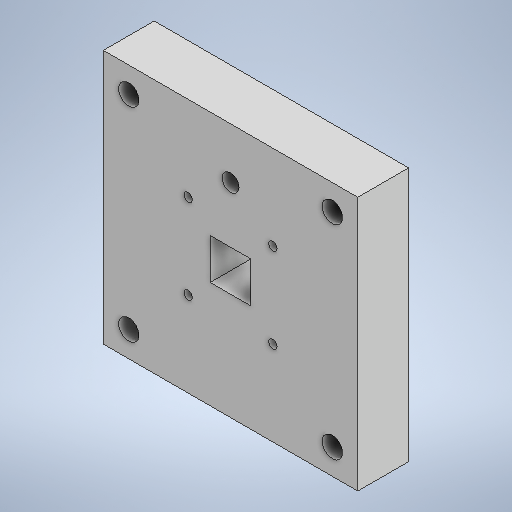
# Autodesk Inventor part: led_cnc
Saved by Autodesk Inventor 2025.1 (Build 291241000, 241)
## iProperties
Created: 2024-10-23
Part Number: led_cnc
Material: Ogólny
Document SubType Name: Modeling
Designer: PC
Density: 1 g/cm^3
Appearance: Domyślna
Author: PC
Autodesk Inventor part; units mm, degrees
ref_plane "YZ Plane" through (0, 0, 0) normal (1, 0, 0) x (0, 1, 0)
ref_plane "XZ Plane" through (0, 0, 0) normal (0, 1, 0) x (-1, 0, 0)
ref_plane "XY Plane" through (0, 0, 0) normal (0, 0, 1) x (1, 0, 0)
sketch "Szkic1" plane through (0, 0, 0) normal (0, 1, 0) x (-1, 0, 0)
  point P0 (0, 0)
sketch "Szkic2" plane through (0, 0, 0) normal (0, 0, 1) x (1, 0, 0)
  line L0 (-37.5, 37.5) -> (37.5, 37.5)
  line L1 (37.5, 37.5) -> (37.5, -37.5)
  line L2 (37.5, -37.5) -> (-37.5, -37.5)
  line L3 (-37.5, -37.5) -> (-37.5, 37.5)
  line L4 (-37.5, 37.5) -> (37.5, -37.5) construction
  line L5 (37.5, 37.5) -> (-37.5, -37.5) construction
  line L6 (-30, -30) -> (30, -30) construction
  line L7 (30, -30) -> (30, 30) construction
  line L8 (30, 30) -> (-30, 30) construction
  line L9 (-30, 30) -> (-30, -30) construction
  line L10 (-30, -30) -> (30, 30) construction
  line L11 (30, -30) -> (-30, 30) construction
  circle A0 centre (30, 30) radius 3
  circle A1 centre (30, -30) radius 3
  circle A2 centre (-30, 30) radius 3
  circle A3 centre (-30, -30) radius 3
  line L12 (-12.5, 12.5) -> (12.5, 12.5) construction
  line L13 (12.5, 12.5) -> (12.5, -12.5) construction
  line L14 (12.5, -12.5) -> (-12.5, -12.5) construction
  line L15 (-12.5, -12.5) -> (-12.5, 12.5) construction
  line L16 (-12.5, 12.5) -> (12.5, -12.5) construction
  line L17 (12.5, 12.5) -> (-12.5, -12.5) construction
  circle A4 centre (12.5, 12.5) radius 1.25
  circle A5 centre (12.5, -12.5) radius 1.25
  circle A6 centre (-12.5, -12.5) radius 1.25
  circle A7 centre (-12.5, 12.5) radius 1.25
  line L18 (-6, -6) -> (6, -6)
  line L19 (6, -6) -> (6, 6)
  line L20 (6, 6) -> (-6, 6)
  line L21 (-6, 6) -> (-6, -6)
  line L22 (-6, -6) -> (6, 6) construction
  line L23 (6, -6) -> (-6, 6) construction
  circle A8 centre (0, 22.5) radius 2.5
  point P0 (0, 0)
  point P1 (0, 37.5)
  dimension "d0" = 75
  dimension "d1" = 60
  dimension "d2" = 6
  dimension "d3" = 25
  dimension "d4" = 2.5
  dimension "d5" = 12
  dimension "d6" = 5
  dimension "d7" = 15
  constraints: 48 end point, 9 centre point, 9 midpoint, 8 coincident, 8 parallel, 8 perpendicular, 6 equal radius, 4 horizontal, 1 vertical alignment
  measures "d0" distance of L0.start L0.end
  measures "d1" distance of L8.end L7.end
  measures "d2" diameter of A0
  measures "d3" distance of L13.end L14.end
  measures "d4" diameter of A4
  measures "d5" distance of L20.end L19.end
  measures "d6" diameter of A8
  measures "d7" distance from line of L0 A8.centre
extrude "Wyciągnięcie proste1" add sketch "Szkic2" along normal blind 15
